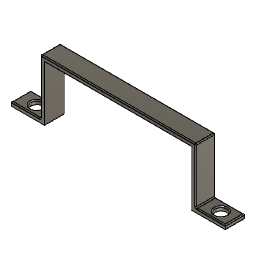
model (Autodesk Fusion 360 design; units mm, degrees)
Autodesk Fusion 360 part; units mm, degrees
box "BoxPrimitive1" add length 10 width 75.25 height 2 placed x (0, -1, 0) y (1, 0, 0) z (0, 0, 1) at (0, 0, 0)
box "BoxPrimitive2" add length 30.25 width 10 height 2 placed x (0, 0, -1) y (0, -1, 0) z (-1, 0, 0) at (0, 0, 2)
box "BoxPrimitive3" add length 30.25 width 10 height 2 placed x (0, 0, -1) y (0, 1, 0) z (1, 0, 0) at (75.25, -10, 2)
box "BoxPrimitive4" add length 2 width 10 height 15 placed x (0, 0, 1) y (0, 1, 0) z (-1, 0, 0) at (-2, -10, -28.25)
box "BoxPrimitive5" add length 2 width 10 height 15 placed x (0, 0, 1) y (0, -1, 0) z (1, 0, 0) at (77.25, 0, -28.25)
hole "Hole1" at (-9.0015, -4.9712, -26.25) direction (0, 0, -1) diameter 6 depth 10 tip angle 118
hole "Hole2" at (84.995, -4.9776, -26.25) direction (0, 0, -1) diameter 6 depth 10 tip angle 118
fillet "Fillet1" radius 0.5 5 faces at (-15.331, -5.0651, -26.25) (78.8345, -5.0673, -26.25) (24.4167, -6.6667, 2) (77.25, -6.6667, -7.4167) (-2, -3.3333, -7.4167)
